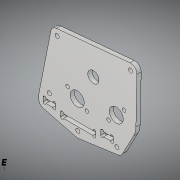
# Autodesk Inventor part: 脚モーターマウント
Saved by Autodesk Inventor 2019 (Build 230136000, 136)
## iProperties
Created: 2019-11-14
Part Number: 脚モーターマウント
Material: アルミニウム 2014-T4
Document SubType Name: Modeling
Designer: tanjihayato
Density: 2.8 g/cm^3
Appearance: サテン
Mass: 29.1091 g
Surface Area: 85.1405 cm^2
Volume: 10.3961 cm^3
Author: tanjihayato
Autodesk Inventor part; units mm, degrees
ref_plane "YZ Plane" through (0, 0, 0) normal (1, 0, 0) x (0, 1, 0)
ref_plane "XZ Plane" through (0, 0, 0) normal (0, 1, 0) x (-1, 0, 0)
ref_plane "XY Plane" through (0, 0, 0) normal (0, 0, 1) x (1, 0, 0)
sketch "スケッチ1" plane through (0, 0, 0) normal (0, 0, 1) x (1, 0, 0)
  circle A0 centre (0, 0) radius 18
  circle A1 centre (-35.3982, 10.7044) radius 1.5
  line L0 (-33.8465, 6.7744) -> (-39.6634, 9.2696)
  arc A2 (-31.9879, 5.2949) -> (-33.8465, 6.7744) centre (-35.6204, 2.6388) ccw
  line L1 (-18.0583, -13.7557) -> (-31.9879, 5.2949)
  arc A3 (-17.339, -17.5569) -> (-18.0583, -13.7557) centre (-21.6908, -16.4118) ccw
  line L2 (-17.339, -17.5569) -> (-23.8868, -42.4405)
  line L3 (21.0739, -11.4259) -> (29.592, -35.7057)
  arc A4 (21.5077, -7.5456) -> (21.0739, -11.4259) centre (25.3202, -9.9362) ccw
  line L4 (34.045, 12.4488) -> (21.5077, -7.5456)
  arc A5 (36.6836, 14.4025) -> (34.045, 12.4488) centre (37.8575, 10.0583) ccw
  line L5 (40.7974, 15.5141) -> (36.6836, 14.4025)
  circle A6 centre (36.7736, 17.5344) radius 1.5
  circle A7 centre (25.6508, -33.5339) radius 1.5
  circle A8 centre (-20.132, -39.9603) radius 1.5
  arc A9 (-23.8868, -42.4405) -> (-19.5065, -44.4166) centre (-20.132, -39.9603) ccw
  line L6 (-19.5065, -44.4166) -> (26.2763, -37.9902)
  arc A10 (26.2763, -37.9902) -> (29.592, -35.7057) centre (25.6508, -33.5339) ccw
  circle A11 centre (27.3908, 10.6821) radius 1.5
  arc A12 (-36.1544, 15.1404) -> (-39.6634, 9.2696) centre (-35.3982, 10.7044) ccw
  arc A13 (40.7942, 15.5132) -> (36.6479, 22.0326) centre (36.7736, 17.5344) ccw
  arc A14 (-0.5868, 20.9918) -> (-3.5285, 20.7014) centre (0, 0) ccw
  line L7 (-36.1544, 15.1404) -> (-3.5285, 20.7014)
  line L8 (-0.5868, 20.9918) -> (36.6479, 22.0326)
  circle A15 centre (14, -17.4118) radius 14 construction
  circle A16 centre (-14, -17.4118) radius 14 construction
  line L9 (-170.6512, -31.4118) -> (202.8656, -31.4118)
  circle A17 centre (-11.0721, -38.6885) radius 3
  circle A18 centre (16.7367, -34.7851) radius 3
  circle A19 centre (26.4774, 17.2466) radius 3
  circle A20 centre (-25.8354, 12.3344) radius 3
  circle A21 centre (0, 0) radius 20.55 construction
  circle A22 centre (-25.8354, 12.3344) radius 1.5
  circle A23 centre (26.4774, 17.2466) radius 1.5
  circle A24 centre (16.7367, -34.7851) radius 1.5
  circle A25 centre (-11.0721, -38.6885) radius 1.5
  circle A26 centre (-11.0721, -38.6885) radius 4.5
  circle A27 centre (16.7367, -34.7851) radius 4.5
  circle A28 centre (26.4774, 17.2466) radius 4.5
  circle A29 centre (-25.8354, 12.3344) radius 4.5
  line L10 (32.7821, 19.6122) -> (19.0889, -6.6924)
  line L11 (-15.7064, -12.7325) -> (-31.5648, 13.0613)
  line L12 (-15.6358, -40.1451) -> (-14.6718, -16.7004)
  line L13 (18.3467, -10.7856) -> (21.1838, -34.078)
  circle A30 centre (0, 0) radius 4
  circle A31 centre (-25.8354, 12.3344) radius 1.5
  circle A32 centre (26.4774, 17.2466) radius 1.5
  circle A33 centre (16.7367, -34.7851) radius 1.5
  circle A34 centre (-11.0721, -38.6885) radius 1.5
  circle A35 centre (14, -17.4118) radius 14 construction
  circle A36 centre (-14, -17.4118) radius 14 construction
  circle A37 centre (0, 0) radius 4
  arc A38 (-26.2561, 16.8147) -> (-29.9839, 14.078) centre (-25.8354, 12.3344) ccw
  arc A39 (30.9006, 16.4185) -> (26.0567, 21.7269) centre (26.4774, 17.2466) ccw
  arc A40 (17.3622, -39.2414) -> (21.1599, -35.6132) centre (16.7367, -34.7851) ccw
  arc A41 (-12.1183, -43.0652) -> (-10.4466, -43.1449) centre (-11.0721, -38.6885) ccw
  circle A42 centre (-14, -17.4118) radius 5
  circle A43 centre (14, -17.4118) radius 5
  circle A44 centre (0, 0) radius 22.3421 construction
  line L14 (-30.3415, -4.2724) -> (0, -28.6685) construction
  line L15 (0, -28.6685) -> (32.9859, -2.1461) construction
  circle A45 centre (-14, -17.4118) radius 8 construction
  circle A46 centre (14, -17.4118) radius 8 construction
  circle A47 centre (-20.2346, -12.3988) radius 1.3
  circle A48 centre (-7.7654, -22.4248) radius 1.3
  circle A49 centre (7.7654, -22.4248) radius 1.3
  circle A50 centre (20.2346, -12.3988) radius 1.3
  line L16 (-170.6512, -31.4118) -> (202.8656, -31.4118)
  line L17 (-42.4, -28.4118) -> (-37.6, -28.4118)
  line L18 (-35.5, -28.4118) -> (-35.5, -31.4118)
  line L19 (-37.6, -31.4118) -> (-42.4, -31.4118)
  line L20 (-44.5, -31.4118) -> (-44.5, -28.4118)
  line L21 (-2.4, -28.4118) -> (2.4, -28.4118)
  line L22 (4.5, -28.4118) -> (4.5, -31.4118)
  line L23 (2.4, -31.4118) -> (-2.4, -31.4118)
  line L24 (-4.5, -31.4118) -> (-4.5, -28.4118)
  line L25 (-30.4, -31.4118) -> (-9.6, -31.4118)
  line L26 (-7.5, -31.4118) -> (-7.5, -34.4118)
  line L27 (-9.6, -34.4118) -> (-30.4, -34.4118)
  line L28 (-32.5, -34.4118) -> (-32.5, -31.4118)
  arc A51 (-42.4, -28.4118) -> (-44.5, -28.4118) centre (-43.45, -28.4118) ccw
  arc A52 (-35.5, -28.4118) -> (-37.6, -28.4118) centre (-36.55, -28.4118) ccw
  arc A53 (-44.5, -31.4118) -> (-42.4, -31.4118) centre (-43.45, -31.4118) ccw
  arc A54 (-37.6, -31.4118) -> (-35.5, -31.4118) centre (-36.55, -31.4118) ccw
  arc A55 (-30.4, -31.4118) -> (-32.5, -31.4118) centre (-31.45, -31.4118) ccw
  arc A56 (-32.5, -34.4118) -> (-30.4, -34.4118) centre (-31.45, -34.4118) ccw
  arc A57 (-7.5, -31.4118) -> (-9.6, -31.4118) centre (-8.55, -31.4118) ccw
  arc A58 (-9.6, -34.4118) -> (-7.5, -34.4118) centre (-8.55, -34.4118) ccw
  arc A59 (-4.5, -31.4118) -> (-2.4, -31.4118) centre (-3.45, -31.4118) ccw
  arc A60 (-2.4, -28.4118) -> (-4.5, -28.4118) centre (-3.45, -28.4118) ccw
  arc A61 (4.5, -28.4118) -> (2.4, -28.4118) centre (3.45, -28.4118) ccw
  arc A62 (2.4, -31.4118) -> (4.5, -31.4118) centre (3.45, -31.4118) ccw
  circle A63 centre (-40, -23.9118) radius 1.5
  circle A64 centre (-40, -23.9118) radius 4.5 construction
  arc A65 (-35.5, -24.5003) -> (-35.5374, -24.4904) centre (-36.55, -28.4118) ccw
  line L29 (-47.5, -28.4118) -> (-47.5, -31.4118)
  arc A66 (-47.5, -31.4118) -> (-44.3916, -35.3508) centre (-43.45, -31.4118) ccw
  line L30 (-47.1836, -26.8425) -> (-29.9839, 14.078)
  line L31 (-26.2561, 16.8147) -> (26.0567, 21.7269)
  line L32 (30.9006, 16.4185) -> (21.1599, -35.6132)
  line L33 (17.3622, -39.2414) -> (-10.4466, -43.1449)
  line L34 (-44.3916, -35.3508) -> (-12.1183, -43.0652)
  arc A67 (-47.1836, -26.8425) -> (-47.5, -28.4118) centre (-43.45, -28.4118) ccw
  circle A68 centre (-11.4931, -19.1593) radius 4
  circle A69 centre (16.245, -15.3385) radius 4
  dimension "d74" = 9
  dimension "d0" = 36
  dimension "d1" = 9
  dimension "d2" = 9
  dimension "d3" = 3
  dimension "d4" = 6
  dimension "d5" = 6
  dimension "d6" = 6
  dimension "d7" = 6
  dimension "d8" = 3
  dimension "d9" = 3
  dimension "d10" = 3
  dimension "d11" = 3
  dimension "d12" = 9
  dimension "d13" = 9
  dimension "d14" = 9
  dimension "d15" = 9
  dimension "d16" = 8
  dimension "d50" = 3
  dimension "d51" = 3
  dimension "d52" = 3
  dimension "d53" = 3
  dimension "d54" = 10
  dimension "d55" = 10
  dimension "d56" = 3
  dimension "d57" = 3
  dimension "d58" = 2.6
  dimension "d59" = 2.6
  dimension "d60" = 2.6
  dimension "d61" = 2.6
  dimension "d62" = 9
  dimension "d63" = 3
  dimension "d64" = 9
  dimension "d65" = 3
  dimension "d66" = 4.5
  dimension "d67" = 40
  dimension "d68" = 25
  dimension "d69" = 3
  dimension "d70" = 3
  dimension "d71" = 3
  dimension "d72" = 2.1
  dimension "d73" = 3
  dimension "d75" = 4.5
  dimension "d76" = 3
  dimension "d77" = 3
  dimension "d78" = 4.05
  constraints: 70 end point, 68 centre point, 60 point on circle, 34 tangent, 25 point on line, 16 coincident, 11 equal radius, 6 parallel, 4 horizontal, 3 perpendicular, 8 other
  measures "d0" diameter of A0
  measures "d1" diameter of A12
  measures "d2" diameter of A13
  measures "d3" radial gap between concentric circles of A0 A14
  measures "d4" diameter of A17
  measures "d5" diameter of A18
  measures "d6" diameter of A19
  measures "d7" diameter of A20
  measures "d8" diameter of A22
  measures "d9" diameter of A23
  measures "d10" diameter of A24
  measures "d11" diameter of A25
  measures "d12" diameter of A26
  measures "d13" diameter of A27
  measures "d14" diameter of A28
  measures "d15" diameter of A29
  measures "d16" diameter of A30
  measures "d50" radial gap between concentric circles of A31 A38
  measures "d51" radial gap between concentric circles of A32 A39
  measures "d52" radial gap between concentric circles of A33 A40
  measures "d53" radial gap between concentric circles of A34 A41
  measures "d54" diameter of A42
  measures "d55" diameter of A43
  measures "d56" radial gap between concentric circles of A42 A45
  measures "d57" radial gap between concentric circles of A43 A46
  measures "d58" diameter of A47
  measures "d59" diameter of A48
  measures "d60" diameter of A49
  measures "d61" diameter of A50
  measures "d62" distance of L18.end L20.start
  measures "d63" distance of L18.start L18.end
  measures "d64" distance of L22.end L24.start
  measures "d65" distance of L22.start L22.end
  measures "d66" distance from line of L22 point (0, 0)
  measures "d67" distance between parallel lines of L18 L22
  measures "d68" distance of L26.end L28.start
  measures "d69" distance of L26.start L26.end
  measures "d70" distance between parallel lines of L26 L24
  measures "d71" distance between parallel lines of L18 L28
  measures "d72" diameter of A51
  measures "d73" diameter of A63
  measures "d75" distance from line of L18 A63.centre
  measures "d76" distance between parallel lines of L29 L20
  measures "d77" radial gap between concentric circles of A66 A53
  measures "d78" radius of A67
sketch "スケッチ2" plane through (0, 0, 0) normal (0, 0, 1) x (1, 0, 0)
  circle A0 centre (-25.8354, 12.3344) radius 1.5 projected
  circle A1 centre (26.4774, 17.2466) radius 1.5 projected
  circle A2 centre (16.7367, -34.7851) radius 1.5 projected
  circle A3 centre (-11.0721, -38.6885) radius 1.5 projected
  circle A4 centre (14, -17.4118) radius 14 construction
  circle A5 centre (-14, -17.4118) radius 14 construction
  circle A6 centre (0, 0) radius 4 projected
  arc A7 (-26.2561, 16.8147) -> (-30.2492, 13.2111) centre (-25.8354, 12.3344) ccw
  arc A8 (30.9763, 17.1458) -> (26.0567, 21.7269) centre (26.4774, 17.2466) ccw
  arc A9 (17.3622, -39.2414) -> (20.7179, -36.8828) centre (16.7367, -34.7851) ccw
  arc A10 (-12.177, -43.0508) -> (-10.4466, -43.1449) centre (-11.0721, -38.6885) ccw
  circle A11 centre (-14, -17.4118) radius 5
  circle A12 centre (14, -17.4118) radius 5
  circle A13 centre (0, 0) radius 22.3421 construction
  line L0 (-30.3415, -4.2724) -> (0, -28.6685) construction
  line L1 (0, -28.6685) -> (32.9859, -2.1461) construction
  circle A14 centre (-14, -17.4118) radius 8 construction
  circle A15 centre (14, -17.4118) radius 8 construction
  circle A16 centre (-20.2346, -12.3988) radius 1.3
  circle A17 centre (-7.7654, -22.4248) radius 1.3
  circle A18 centre (7.7654, -22.4248) radius 1.3
  circle A19 centre (20.2346, -12.3988) radius 1.3
  line L2 (-33.6846, -30.1593) -> (-28.8846, -30.1593)
  line L3 (-26.7846, -30.1593) -> (-26.7846, -33.1593)
  line L4 (-28.8846, -33.1593) -> (-33.6846, -33.1593)
  line L5 (-35.7846, -33.1593) -> (-35.7846, -30.1593)
  line L6 (7.3154, -30.1593) -> (12.1154, -30.1593)
  line L7 (14.2154, -30.1593) -> (14.2154, -33.1593)
  line L8 (12.1154, -33.1593) -> (7.3154, -33.1593)
  line L9 (5.2154, -33.1593) -> (5.2154, -30.1593)
  line L10 (-21.1846, -33.1593) -> (-0.3846, -33.1593)
  line L11 (1.7154, -33.1593) -> (1.7154, -36.1593)
  line L12 (-0.3846, -36.1593) -> (-21.1846, -36.1593)
  line L13 (-23.2846, -36.1593) -> (-23.2846, -33.1593)
  arc A20 (-33.6846, -30.1593) -> (-35.7846, -30.1593) centre (-34.7346, -30.1593) ccw
  arc A21 (-26.7846, -30.1593) -> (-28.8846, -30.1593) centre (-27.8346, -30.1593) ccw
  arc A22 (-35.7846, -33.1593) -> (-33.6846, -33.1593) centre (-34.7346, -33.1593) ccw
  arc A23 (-28.8846, -33.1593) -> (-26.7846, -33.1593) centre (-27.8346, -33.1593) ccw
  arc A24 (-21.1846, -33.1593) -> (-23.2846, -33.1593) centre (-22.2346, -33.1593) ccw
  arc A25 (-23.2846, -36.1593) -> (-21.1846, -36.1593) centre (-22.2346, -36.1593) ccw
  arc A26 (1.7154, -33.1593) -> (-0.3846, -33.1593) centre (0.6654, -33.1593) ccw
  arc A27 (-0.3846, -36.1593) -> (1.7154, -36.1593) centre (0.6654, -36.1593) ccw
  arc A28 (5.2154, -33.1593) -> (7.3154, -33.1593) centre (6.2654, -33.1593) ccw
  arc A29 (7.3154, -30.1593) -> (5.2154, -30.1593) centre (6.2654, -30.1593) ccw
  arc A30 (14.2154, -30.1593) -> (12.1154, -30.1593) centre (13.1654, -30.1593) ccw
  arc A31 (12.1154, -33.1593) -> (14.2154, -33.1593) centre (13.1654, -33.1593) ccw
  circle A32 centre (-31.2846, -25.6593) radius 1.5
  circle A33 centre (-31.2846, -25.6593) radius 4.5 construction
  line L14 (-38.7846, -30.1593) -> (-38.7846, -33.1593)
  arc A34 (-38.7846, -33.1593) -> (-35.729, -37.0854) centre (-34.7346, -33.1593) ccw
  line L15 (-38.707, -29.3703) -> (-30.2492, 13.2111)
  line L16 (-26.2561, 16.8147) -> (26.0567, 21.7269)
  line L17 (17.3622, -39.2414) -> (-10.4466, -43.1449)
  line L18 (-35.729, -37.0854) -> (-12.177, -43.0508)
  arc A35 (-38.707, -29.3703) -> (-38.7846, -30.1593) centre (-34.7346, -30.1593) ccw
  circle A36 centre (-11.4931, -19.1593) radius 4 construction
  circle A37 centre (16.245, -15.3385) radius 4 construction
  circle A38 centre (-11.4931, -19.1593) radius 5
  circle A39 centre (16.245, -15.3385) radius 5
  line L19 (-26.4603, -10.181) -> (3.9121, -28.4004) construction
  line L20 (3.9121, -28.4004) -> (26.0888, -4.913) construction
  circle A40 centre (-11.4931, -19.1593) radius 8 construction
  circle A41 centre (16.245, -15.3385) radius 8 construction
  circle A42 centre (-18.3534, -15.044) radius 1.3
  circle A43 centre (-4.6327, -23.2746) radius 1.3
  circle A44 centre (10.7528, -21.1553) radius 1.3
  circle A45 centre (21.7373, -9.5217) radius 1.3
  circle A46 centre (-11.4931, -19.1593) radius 14
  arc A47 (28.6309, -21.8646) -> (30.2415, -15.6521) centre (16.245, -15.3385) ccw
  circle A48 centre (16.7367, -34.7851) radius 3
  line L21 (30.9763, 17.1458) -> (30.2415, -15.6521)
  line L22 (28.6309, -21.8646) -> (20.7179, -36.8828)
  circle A49 centre (-11.0721, -38.6885) radius 3
  dimension "d91" = 6
  dimension "d17" = 3
  dimension "d18" = 3
  dimension "d19" = 3
  dimension "d20" = 3
  dimension "d21" = 10
  dimension "d22" = 10
  dimension "d23" = 3
  dimension "d24" = 3
  dimension "d25" = 2.6
  dimension "d26" = 2.6
  dimension "d27" = 2.6
  dimension "d28" = 2.6
  dimension "d29" = 9
  dimension "d30" = 3
  dimension "d31" = 9
  dimension "d32" = 3
  dimension "d35" = 25
  dimension "d36" = 3
  dimension "d37" = 3.5
  dimension "d38" = 3.5
  dimension "d39" = 2.1
  dimension "d40" = 3
  dimension "d42" = 9
  dimension "d44" = 4.5
  dimension "d45" = 3
  dimension "d46" = 3
  dimension "d47" = 4.05
  dimension "d79" = 10
  dimension "d80" = 10
  dimension "d81" = 3
  dimension "d82" = 3
  dimension "d83" = 2.6
  dimension "d84" = 2.6
  dimension "d85" = 2.6
  dimension "d86" = 2.6
  dimension "d89" = 28
  dimension "d90" = 28
  dimension "d92" = 50
  dimension "d93" = 6
  constraints: 46 end point, 46 point on circle, 39 centre point, 26 tangent, 24 point on line, 11 equal radius, 10 coincident, 6 parallel, 3 horizontal, 3 perpendicular, 2 collinear, 10 other
  measures "d17" radial gap between concentric circles of A0 A7
  measures "d18" radial gap between concentric circles of A1 A8
  measures "d19" radial gap between concentric circles of A2 A9
  measures "d20" radial gap between concentric circles of A3 A10
  measures "d21" diameter of A11
  measures "d22" diameter of A12
  measures "d23" radial gap between concentric circles of A11 A14
  measures "d24" radial gap between concentric circles of A12 A15
  measures "d25" diameter of A16
  measures "d26" diameter of A17
  measures "d27" diameter of A18
  measures "d28" diameter of A19
  measures "d29" distance of L3.end L5.start
  measures "d30" distance of L3.start L3.end
  measures "d31" distance of L7.end L9.start
  measures "d32" distance of L7.start L7.end
  measures "d35" distance of L11.end L13.start
  measures "d36" distance of L11.start L11.end
  measures "d37" distance between parallel lines of L11 L9
  measures "d38" distance between parallel lines of L3 L13
  measures "d39" diameter of A20
  measures "d40" diameter of A32
  measures "d42" diameter of A33
  measures "d44" distance from line of L3 A32.centre
  measures "d45" distance between parallel lines of L14 L5
  measures "d46" radial gap between concentric circles of A34 A22
  measures "d47" radius of A35
  measures "d79" diameter of A38
  measures "d80" diameter of A39
  measures "d81" radial gap between concentric circles of A38 A40
  measures "d82" radial gap between concentric circles of A39 A41
  measures "d83" diameter of A42
  measures "d84" diameter of A43
  measures "d85" diameter of A44
  measures "d86" diameter of A45
  measures "d89" diameter of A46
  measures "d90" diameter of A47
  measures "d92" distance between parallel lines of L5 L7
  measures "d93" diameter of A49
extrude "押し出し1" add sketch "スケッチ2" along normal blind 3 contours L16 A8 L21 A47 L22 A9 L17 A10 L18 A34 L14 A35 L15 A7 | A11 A38 | A11 A38 A17 | A38 A11 A42 | A42 A11 | A11 A42 | A38 A17 | A17 A38 | A12 A39 | A12 A39 A19 | A39 A12 A44 | A44 A12 | A12 A44 | A39 A19 | A19 A39 | A16 | A18 | A48 A31 | A46 | L12 A49 | A43 | A45 picked at (19.1924, -35.1468) picked at (-11.0118, -36.506)
extrude "押し出し2" cut sketch "スケッチ2" along normal blind 10 contours A11 A38 | A11 A38 A17 | A42 A11 | A11 A42 | A17 A38 | A12 A39 | A12 A39 A19 | A44 A12 | A12 A44 | A39 A19 | A43 | A45 picked at (-8.0787, -22.1504) picked at (19.8993, -12.6458)
equation "\"d71\" = d70"
equation "\"d38\" = d37"
